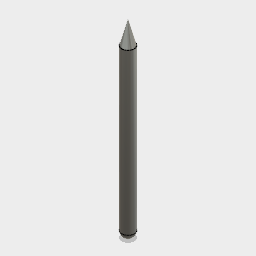
pencil (Autodesk Fusion 360 design; units mm, degrees)
Autodesk Fusion 360 part; units mm, degrees
cylinder "圆柱体基本要素1" add diameter 8 height 100 placed x (1, 0, 0) y (0, 0, -1) z (0, 1, 0) at (10, 0, 10) makes body 1
sphere "球体基本要素1" add diameter 8 placed x (1, 0, 0) y (0, 0, -1) z (0, 1, 0) at (55, 0, 20) separate body makes body 2
move_body "对齐1" bodies 2 to x (1, 0, 0) y (0, 0, 1) z (0, -1, 0) at (-45, 20, 10)
sketch "草图3" plane through (0, 0, 0) normal (0, 0, 1) x (1, 0, 0)
  line L0 (100, 30) -> (100, 45)
  line L1 (100, 45) -> (104, 45)
  line L2 (104, 45) -> (100, 30)
  dimension "d4" = 15
  dimension "d5" = 4
  measures "d4" distance of L0.start L0.end
  measures "d5" distance of L0.end L1.end
revolve "旋转1" add sketch "草图3" angle 360 about axis through (104, 45, 0) along (-0.25766265, -0.96623494, 0) separate body contours L0 L1 L2 picked at (101.333333, 40) makes body 3
move_body "对齐2" bodies 3 to x (-0.96623494, -0.25766265, 0) y (0.25766265, -0.96623494, 0) z (0, 0, 1) at (98.893614, 169.246837, 10)
combine "合并1" operation add target body 3 tool bodies 2 1
